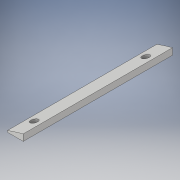
# Autodesk Inventor part: podkladka2
Saved by Autodesk Inventor 2019.4 (Build 234330000, 330)
## iProperties
Created: 2019-06-02
Part Number: podkladka2
Material: Ogólne
Document SubType Name: Modeling
Designer: Esterka
Density: 1 g/cm^3
Appearance: Domyślne
Author: Esterka
Autodesk Inventor part; units mm, degrees
ref_plane "YZ Plane" through (0, 0, 0) normal (1, 0, 0) x (0, 1, 0)
ref_plane "XZ Plane" through (0, 0, 0) normal (0, 1, 0) x (-1, 0, 0)
ref_plane "XY Plane" through (0, 0, 0) normal (0, 0, 1) x (1, 0, 0)
sketch "Sketch1" plane through (0, 0, 0) normal (0, 0, 1) x (1, 0, 0)
  line L0 (-5.4083, 6.8084) -> (-5.4083, 5.8084)
  line L1 (-5.4083, 5.8084) -> (4.5917, 5.8084)
  line L2 (4.5917, 5.8084) -> (4.5917, 9.943)
  arc A0 (4.5917, 9.943) -> (-5.4083, 6.8084) centre (35.0917, -104.875) ccw
  dimension "d24" = 1
  constraints: 6 end point, 2 point on circle, 1 centre point, 1 perpendicular, 1 vertical
  measures "d24" distance of L0.start L0.end
extrude "Extrusion1" add sketch "Sketch1" along normal blind 95
sketch "Sketch4" plane through (-5.4083, 5.8084, 0) normal (0, -1, 0) x (1, 0, 0)
  line L0 (0, 95) -> (10, 95) projected
  line L1 (0, 0) -> (0, 95) projected
  line L2 (0, 0) -> (10, 0) projected
  point P0 (5.4083, 0)
  point P1 (5, 12)
  point P2 (5, 83)
  dimension "d25" = 12
  dimension "d26" = 5
  dimension "d27" = 12
  dimension "d28" = 5
  measures "d25" distance from line of L0 point (5, 83)
  measures "d26" distance from line of L1 point (5, 83)
  measures "d27" distance from line of L2 point (5, 12)
  measures "d28" distance from line of L1 point (5, 12)
hole "Hole2" at (-0.4083, 5.8084, 12) at (-0.4083, 5.8084, 83) direction (0, 1, 0) diameter 4.5 depth 8 tip angle 118 clearance for "Countersunk Flat Head Screw ISO 2009/7046" size "M4" standard "ISO"
body "Solid1"
